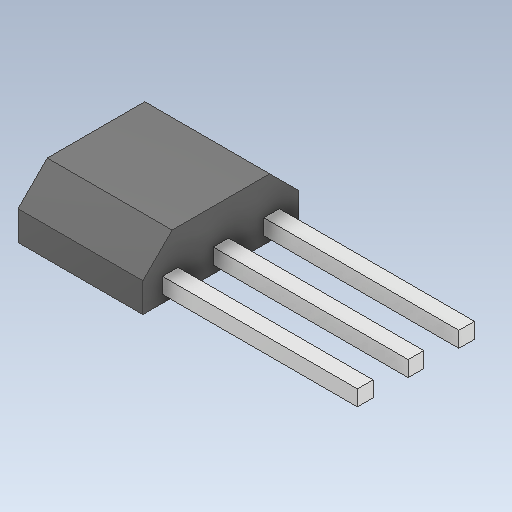
# Autodesk Inventor part: 08-04-02-008_hallSensor
Saved by Autodesk Inventor 2020 (Build 240168000, 168)
## iProperties
Created: 2021-08-28
Part Number: 08-04-02-008_hallSensor
Material: ABS-Kunststoff(1)
Document SubType Name: Modeling
Designer: Eric
Density: 1.06 g/cm^3
Appearance: Glatt - Weiß(1)
Author: Eric
Autodesk Inventor part; units mm, degrees
ref_plane "YZ Plane" through (0, 0, 0) normal (1, 0, 0) x (0, 1, 0)
ref_plane "XZ Plane" through (0, 0, 0) normal (0, 1, 0) x (-1, 0, 0)
ref_plane "XY Plane" through (0, 0, 0) normal (0, 0, 1) x (1, 0, 0)
sketch "Skizze1" plane through (0, 0, 0) normal (1, 0, 0) x (0, 1, 0)
  line L0 (0, 0) -> (0, 4)
  line L1 (0, 4) -> (0.75, 4)
  line L2 (0.75, 4) -> (1.5, 3.25)
  line L3 (1.5, 3.25) -> (1.5, 0.75)
  line L4 (1.5, 0.75) -> (0.75, 0)
  line L5 (0.75, 0) -> (0, 0)
  point P0 (1.5, 2)
  point P1 (0, 2)
  dimension "d0" = 4
  dimension "d1" = 1.5
  dimension "d2" = 0.75
  dimension "d3" = 45
  constraints: 12 end point, 2 equal length, 2 midpoint, 2 perpendicular, 1 horizontal alignment, 1 parallel, 1 vertical
  measures "d0" distance of L0.start L0.end
  measures "d1" distance between parallel lines of L0 L3
  measures "d2" distance of L0.end L1.end
  measures "d3" angle of L1 L2
extrude "Extrusion1" add sketch "Skizze1" along normal blind 3.2
sketch "Skizze2" plane through (3.2, 0, 0) normal (1, 0, 0) x (0, 0, -1)
  line L0 (-3.1, 0.2) -> (-3.5, 0.2)
  line L1 (-3.5, 0.2) -> (-3.5, 0.6)
  line L2 (-3.5, 0.6) -> (-3.1, 0.6)
  line L3 (-3.1, 0.6) -> (-3.1, 0.2)
  line L4 (-1.8, 0.6) -> (-2.2, 0.6)
  line L5 (-2.2, 0.6) -> (-2.2, 0.2)
  line L6 (-2.2, 0.2) -> (-1.8, 0.2)
  line L7 (-1.8, 0.2) -> (-1.8, 0.6)
  line L8 (-0.9, 0.6) -> (-0.5, 0.6)
  line L9 (-0.5, 0.6) -> (-0.5, 0.2)
  line L10 (-0.5, 0.2) -> (-0.9, 0.2)
  line L11 (-0.9, 0.2) -> (-0.9, 0.6)
  line L12 (-3.5, 0.4) -> (-0.5, 0.4) construction
  line L13 (-0.75, 1.5) -> (-3.25, 1.5) projected
  point P0 (0, 0)
  point P1 (-2, 0.4)
  point P2 (-2, 0.6)
  point P3 (-2.2, 0.4)
  point P4 (-2, 1.5)
  dimension "d6" = 0.4
  dimension "d7" = 3
  dimension "d8" = 0.9
  constraints: 26 end point, 6 midpoint, 6 parallel, 5 equal length, 4 horizontal, 3 perpendicular, 2 vertical alignment, 1 horizontal alignment
  measures "d6" distance of L0.end L1.end
  measures "d7" distance between parallel lines of L9 L1
  measures "d8" distance between parallel lines of L13 L4
extrude "Extrusion2" add sketch "Skizze2" along normal blind 5
